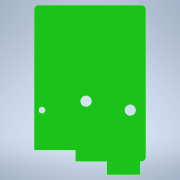
# Autodesk Inventor part: Pared_caja_reduccion_MDF
Saved by Autodesk Inventor 2022 (Build 260153000, 153)
## iProperties
Created: 2022-02-27
Part Number: Pared_caja_reduccion_MDF
Material: Generic
Document SubType Name: Modeling
Designer: Home
Density: 1 g/cm^3
Appearance: Dark Green
Author: Home
Autodesk Inventor part; units mm, degrees
ref_plane "YZ Plane" through (0, 0, 0) normal (1, 0, 0) x (0, 1, 0)
ref_plane "XZ Plane" through (0, 0, 0) normal (0, 1, 0) x (-1, 0, 0)
ref_plane "XY Plane" through (0, 0, 0) normal (0, 0, 1) x (1, 0, 0)
sketch "Sketch2" plane through (0, 0, 0) normal (0, 1, 0) x (-1, 0, 0)
  line L0 (25, -35) -> (-25, -35)
  line L1 (-25, -35) -> (-25, 35)
  line L2 (25, 30) -> (25, -35)
  line L3 (25, -35) -> (-25, 35) construction
  line L4 (-25, -35) -> (25, 35) construction
  line L5 (12, 35) -> (-3, 35)
  line L6 (6.5, 35) -> (12, 35)
  line L7 (-3, 35) -> (-25, 35)
  line L8 (25, 35) -> (6.5, 35)
  line L9 (6.5, 35) -> (6.5, 30)
  line L10 (6.5, 30) -> (25, 30)
  line L11 (25, 30) -> (25, 35)
  line L12 (-22.5, 35) -> (-7.5, 35)
  line L13 (-7.5, 35) -> (-7.5, 41)
  line L14 (-7.5, 41) -> (-22.5, 41)
  line L15 (-22.5, 41) -> (-22.5, 35)
  point P0 (0, 0)
  point P1 (0, 0)
  point P2 (-7.5, 35)
  dimension "d0" = 50
  dimension "d1" = 70
  dimension "d16" = 18.5
  dimension "d17" = 5
  dimension "d58" = 2.5
  dimension "d59" = 15
  dimension "d60" = 6
  constraints: 32 end point, 6 horizontal, 5 parallel, 3 midpoint, 3 perpendicular, 1 point on line
  measures "d0" distance of L1.end L4.end
  measures "d1" distance of L0.end L1.end
  measures "d16" distance of L2.start L9.end
  measures "d17" distance of L6.start L9.end
  measures "d58" distance between parallel lines of L1 L15
  measures "d59" distance of L13.end L14.end
  measures "d60" distance of L12.end L13.end
extrude "Extrusion3" add sketch "Sketch2" along normal blind 6 contours L0 L1 L7 L5 L9 L10 L2 | L15 L14 L13 L7
fillet "Fillet1" radius 2 3 edges at (25, 3, -35) (-25, 3, -35) (25, 3, 35)
sketch "Sketch4" plane through (0, 6, 0) normal (0, 1, 0) x (1, 0, 0)
  circle A0 centre (-1.75, -8) radius 2.5
  line L0 (25, -33) -> (25, 33) projected
  circle A1 centre (-21.5, -12) radius 1.5
  line L1 (-25, 33) -> (-25, -30) projected
  circle A2 centre (18, -12) radius 2.5
  line L2 (-6.5, -35) -> (7.5, -35) projected
  point P0 (0, 0)
  dimension "d31" = 5
  dimension "d34" = 3
  dimension "d41" = 5
  dimension "d44" = 19.75
  dimension "d45" = 19.75
  dimension "d46" = 7
  dimension "d61" = 23
  dimension "d62" = 27
  dimension "d63" = 23
  constraints: 3 centre point
  measures "d31" diameter of A0
  measures "d34" diameter of A1
  measures "d41" diameter of A2
  measures "d44" horizontal distance of A0.centre A2.centre
  measures "d45" horizontal distance of A1.centre A0.centre
  measures "d46" distance from line of L0 A2.centre
  measures "d61" distance from line of L2 A2.centre
  measures "d62" distance from line of L2 A0.centre
  measures "d63" distance from line of L2 A1.centre
extrude "Extrusion10" cut sketch "Sketch4" against normal through all
body "Solid3"
